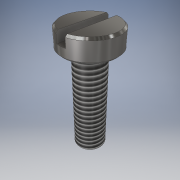
# Autodesk Inventor part: Bolt-M3x10
Saved by Autodesk Inventor 2018 (Build 220112000, 112)
## iProperties
Created: 2020-04-17
Part Number: Bolt-M3x10
Material: Ocel, vysokopevnostní, nízkolegovaná
Document SubType Name: Modeling
Designer: Jozko Mrkvicka
Density: 7.85 g/cm^3
Appearance: Ocel – leštěná
Mass: 0.878596 g
Surface Area: 1.79962 cm^2
Volume: 0.111923 cm^3
Author: Jozko Mrkvicka
Autodesk Inventor part; units mm, degrees
ref_plane "YZ Plane" through (0, 0, 0) normal (1, 0, 0) x (0, 1, 0)
ref_plane "XZ Plane" through (0, 0, 0) normal (0, 1, 0) x (-1, 0, 0)
ref_plane "XY Plane" through (0, 0, 0) normal (0, 0, 1) x (1, 0, 0)
sketch "Náčrt1" plane through (0, 0, 0) normal (0, 0, 1) x (1, 0, 0)
  circle A0 centre (0, 0) radius 2.75
  dimension "d0" = 5.5
  constraints: 1 centre point, 1 coincident
  measures "d0" diameter of A0
extrude "Vysunutí1" add sketch "Náčrt1" along normal blind 2
chamfer "Zkosení1" distance 0.2 angle 45 1 edges at (-2.75, 0, 2)
chamfer "Zkosení2" distance 0.2 angle 45 1 edges at (-2.75, 0, 0)
sketch "Náčrt2" plane through (0, 0, 2) normal (0, 0, 1) x (1, 0, 0)
  line L0 (-0.6097, -6) -> (0.3903, -6)
  line L1 (0.3903, -6) -> (0.3903, 6)
  line L2 (0.3903, 6) -> (-0.6097, 6)
  line L3 (-0.6097, 6) -> (-0.6097, -6)
  line L4 (-0.6097, -6) -> (0.3903, 6) construction
  line L5 (0.3903, -6) -> (-0.6097, 6) construction
  point P0 (0, 0)
  point P1 (-0.1097, 0)
  dimension "d9" = 1
  constraints: 12 end point, 2 midpoint, 2 parallel, 1 horizontal, 1 perpendicular
  measures "d9" distance of L2.end L1.end
extrude "Vysunutí2" cut sketch "Náčrt2" against normal blind 1
sketch "Náčrt3" plane through (0, 0, 0) normal (0, 0, -1) x (-1, 0, 0)
  circle A0 centre (0, 0) radius 1.5
  dimension "d12" = 3
  constraints: 1 centre point, 1 coincident
  measures "d12" diameter of A0
extrude "Vysunutí3" add sketch "Náčrt3" along normal blind 10
chamfer "Zkosení3" distance 0.2 angle 45 1 edges at (1.5, 0, -10)
thread "Závit1" size "M3x0.5" class "6g" standard "ANSI Metric M Profile" full length
